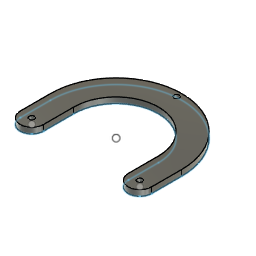
Design A Clamp (Autodesk Fusion 360 design; units mm, degrees)
Autodesk Fusion 360 part; units mm, degrees
sketch "Sketch1" plane through (0, 0, 0) normal (0, 0, 1) x (1, 0, 0)
  line L0 (68.385, 0) -> (68.385, -31.04)
  line L1 (44.135, 0) -> (44.135, -31.04)
  line L2 (68.385, -31.525) -> (68.385, -31.04)
  line L3 (44.135, -31.525) -> (44.135, -31.04)
  line L4 (-68.385, 0) -> (-68.385, -31.04)
  line L5 (-44.135, 0) -> (-44.135, -31.04)
  line L6 (-68.385, -31.525) -> (-68.385, -31.04)
  line L7 (-44.135, -31.525) -> (-44.135, -31.04)
  arc A0 (44.135, 0) -> (-44.135, 0) centre (0, 0) ccw
  arc A1 (68.385, 0) -> (-68.385, 0) centre (0, 0) ccw
  arc A2 (44.135, -31.525) -> (68.385, -31.525) centre (56.26, -31.525) ccw
  arc A3 (-68.385, -31.525) -> (-44.135, -31.525) centre (-56.26, -31.525) ccw
  constraint vertical L0
extrude "Extrude5" add sketch "Sketch1" along normal blind 6
sketch "Sketch4" plane through (0, 0, 0) normal (0, 0, 1) x (1, 0, 0)
sketch "Sketch5" plane through (0, 0, 6) normal (0, 0, 1) x (-1, 0, 0)
  arc A0 (-68.385, 0) -> (68.385, 0) centre (0, 0) ccw
  line L0 (68.385, 0) -> (68.385, 31.525)
  arc A1 (68.385, 31.525) -> (44.135, 31.525) centre (56.26, 31.525) ccw
  line L1 (44.135, 31.525) -> (44.135, 0)
  arc A2 (-44.135, 0) -> (44.135, 0) centre (0, 0) ccw
  line L2 (-44.135, 0) -> (-44.135, 31.525)
  arc A3 (-44.135, 31.525) -> (-68.385, 31.525) centre (-56.26, 31.525) ccw
  line L3 (-68.385, 31.525) -> (-68.385, 0)
  circle A4 centre (56.26, 31.525) radius 2.75
  circle A5 centre (-56.26, 31.525) radius 2.75
  circle A6 centre (0, -63) radius 2.75
  dimension "d79" = 5.5
  dimension "d80" = 5.5
  dimension "d82" = 5.5
  constraint concentric A3 A5
  constraint coincident A1.centre A4.centre
  measures "d79" diameter of A4
  measures "d80" diameter of A5
  measures "d82" diameter of A6
extrude "Extrude6" cut sketch "Sketch5" against normal blind 6 contours A4 | A5 | A6
